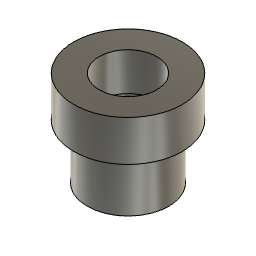
The cap (Autodesk Fusion 360 design; units mm, degrees)
Autodesk Fusion 360 part; units mm, degrees
sketch "Sketch1" plane through (0, 0, 0) normal (0, 0, 1) x (1, 0, 0)
  circle A0 centre (0, 0) radius 5
  circle A1 centre (0, 0) radius 10
  dimension "d1" = 10
  dimension "d2" = 20
  constraint coincident A0.centre A1.centre
  constraint concentric A0 A1
  measures "d1" diameter of A0
  measures "d2" diameter of A1
extrude "Extrude1" add sketch "Sketch1" along normal blind 7.5
sketch "Sketch2" plane through (0, 0, 0) normal (0, 0, 1) x (1, 0, 0)
  circle A0 centre (0, 0) radius 3.05
  circle A1 centre (0, 0) radius 7.5
  dimension "d5" = 6.1
  dimension "d6" = 15
  constraint coincident A0.centre A1.centre
  constraint concentric A0 A1
  measures "d5" diameter of A0
  measures "d6" diameter of A1
extrude "Extrude2" add sketch "Sketch2" against normal blind 10
sketch "草图3" plane through (0, 0, 0) normal (0, 0, 1) x (1, 0, 0)
  circle A0 centre (0, 0) radius 6
  dimension "d9" = 12
  constraint coincident A0.centre origin
  measures "d9" diameter of A0
extrude "拉伸3" cut sketch "草图3" along normal blind 8
sketch "草图4" plane through (0, 0, 0) normal (0, 0, 1) x (1, 0, 0)
  circle A0 centre (0, 0) radius 3.25
  dimension "d12" = 6.5
  constraint coincident A0.centre origin
  measures "d12" diameter of A0
extrude "拉伸4" cut sketch "草图4" against normal blind 10
sketch "草图5" plane through (0, 0, 0) normal (0, 0, 1) x (1, 0, 0)
  circle A0 centre (0, 0) radius 5.75
  circle A1 centre (0, 0) radius 6
  dimension "d15" = 11.5
  constraint coincident A0.centre A1.centre
  measures "d15" diameter of A0
extrude "拉伸5" add sketch "草图5" along normal blind 7.5
sketch "草图6" plane through (0, 0, 0) normal (0, 0, 1) x (1, 0, 0)
  circle A0 centre (0, 0) radius 5.4
  circle A1 centre (0, 0) radius 5.75
  dimension "d18" = 10.8
  dimension "d19" = 11.5
  constraint coincident A0.centre A1.centre
  measures "d18" diameter of A0
  measures "d19" diameter of A1
extrude "拉伸6" add sketch "草图6" along normal blind 7.5
sketch "草图7" plane through (0, 0, 7.5) normal (0, 0, 1) x (-1, 0, 0)
  circle A0 centre (0, 0) radius 5.4
  circle A1 centre (0, 0) radius 10
extrude "拉伸7" add sketch "草图7" against normal blind 7 contours A0
sketch "草图8" plane through (0, 0, 7.5) normal (0, 0, 1) x (-1, 0, 0)
  circle A0 centre (0, 0) radius 10
  circle A1 centre (0, 0) radius 5.3
  dimension "d24" = 10.6
  constraint concentric A0 A1
  measures "d24" diameter of A1
extrude "拉伸8" cut sketch "草图8" against normal blind 7 contours A1
